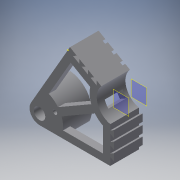
# Autodesk Inventor part: Base_Alpha_V1.1_6mm_
Saved by Autodesk Inventor 2016 (Build 200138000, 138)
## iProperties
Created: 2015-12-07
Part Number: Base_Alpha_V1.1_6mm_
Material: Generic
Document SubType Name: Modeling
Designer: Daniel
Density: 1 g/cm^3
Appearance: Default
Author: Daniel
Autodesk Inventor part; units mm, degrees
ref_plane "YZ Plane" through (0, 0, 0) normal (1, 0, 0) x (0, 1, 0)
ref_plane "XZ Plane" through (0, 0, 0) normal (0, 1, 0) x (-1, 0, 0)
ref_plane "XY Plane" through (0, 0, 0) normal (0, 0, 1) x (1, 0, 0)
sketch "Sketch1" plane through (0, 0, 0) normal (0, 1, 0) x (-1, 0, 0)
  circle A0 centre (103.923, -60) radius 8
  line L0 (24.2487, 14) -> (32.909, 19)
  line L1 (36.3731, 21) -> (45.0333, 26)
  line L2 (48.4974, 28) -> (57.1577, 33)
  line L3 (0, -28) -> (0, -38)
  line L4 (0, -42) -> (0, -52)
  line L5 (0, -56) -> (0, -66)
  line L6 (5.1962, -74) -> (103.923, -74)
  arc A1 (103.923, -74) -> (116.0474, -53) centre (103.923, -60) ccw
  line L7 (116.0474, -53) -> (61.4878, 41.5)
  arc A2 (5.1962, -23.4307) -> (17.6935, 16.2154) centre (0, 0) ccw
  line L8 (5.1962, -23.4307) -> (5.1962, -31)
  line L9 (5.1962, -31) -> (0, -28)
  line L10 (0, -28) -> (0, -38)
  line L11 (0, -38) -> (5.1962, -35)
  line L12 (5.1962, -35) -> (5.1962, -45)
  line L13 (5.1962, -45) -> (0, -42)
  line L14 (0, -42) -> (0, -52)
  line L15 (0, -52) -> (5.1962, -49)
  line L16 (5.1962, -49) -> (5.1962, -59)
  line L17 (5.1962, -59) -> (0, -56)
  line L18 (0, -56) -> (0, -66)
  line L19 (0, -66) -> (5.1962, -63)
  line L20 (5.1962, -63) -> (5.1962, -74)
  line L21 (17.6935, 16.2154) -> (24.2487, 20)
  line L22 (24.2487, 20) -> (24.2487, 14)
  line L23 (24.2487, 14) -> (32.909, 19)
  line L24 (32.909, 19) -> (27.7128, 22)
  line L25 (27.7128, 22) -> (36.3731, 27)
  line L26 (36.3731, 27) -> (36.3731, 21)
  line L27 (36.3731, 21) -> (45.0333, 26)
  line L28 (45.0333, 26) -> (39.8372, 29)
  line L29 (39.8372, 29) -> (48.4974, 34)
  line L30 (48.4974, 34) -> (48.4974, 28)
  line L31 (48.4974, 28) -> (57.1577, 33)
  line L32 (57.1577, 33) -> (51.9615, 36)
  line L33 (51.9615, 36) -> (61.4878, 41.5)
  line L34 (91.0088, -29.6319) -> (60.4256, 23.3397)
  line L35 (60.4256, 23.3397) -> (33.1425, 7.5878)
  arc A3 (31.6247, -12.485) -> (33.1425, 7.5878) centre (0, 0) ccw
  line L36 (31.6247, -12.485) -> (78.1742, -39.3604)
  arc A4 (91.0088, -29.6319) -> (78.1742, -39.3604) centre (103.923, -60) ccw
  line L37 (71.1664, -64) -> (15.1962, -64)
  line L38 (15.1962, -64) -> (15.1962, -30.4151)
  arc A5 (15.1962, -30.4151) -> (26.6247, -21.1453) centre (0, 0) ccw
  line L39 (26.6247, -21.1453) -> (73.1742, -48.0206)
  arc A6 (73.1742, -48.0206) -> (71.1664, -64) centre (103.923, -60) ccw
  line L40 (61.4878, 41.5) -> (116.0474, -53)
  line L41 (61.4878, 41.5) -> (51.9615, 36)
  line L42 (57.1577, 33) -> (51.9615, 36)
  line L43 (57.1577, 33) -> (48.4974, 28)
  line L44 (48.4974, 34) -> (48.4974, 28)
  line L45 (48.4974, 34) -> (39.8372, 29)
  line L46 (45.0333, 26) -> (39.8372, 29)
  line L47 (45.0333, 26) -> (36.3731, 21)
  line L48 (36.3731, 21) -> (36.3731, 27)
  line L49 (36.3731, 27) -> (27.7128, 22)
  line L50 (32.909, 19) -> (27.7128, 22)
  line L51 (32.909, 19) -> (24.2487, 14)
  line L52 (24.2487, 14) -> (24.2487, 20)
  line L53 (24.2487, 20) -> (17.6935, 16.2154)
  line L54 (5.1962, -23.4307) -> (5.1962, -31)
  line L55 (0, -28) -> (5.1962, -31)
  line L56 (0, -28) -> (0, -38)
  line L57 (5.1962, -35) -> (0, -38)
  line L58 (5.1962, -35) -> (5.1962, -45)
  line L59 (0, -42) -> (5.1962, -45)
  line L60 (0, -42) -> (0, -52)
  line L61 (0, -52) -> (5.1962, -49)
  line L62 (5.1962, -49) -> (5.1962, -59)
  line L63 (0, -56) -> (5.1962, -59)
  line L64 (0, -56) -> (0, -66)
  line L65 (5.1962, -63) -> (0, -66)
  line L66 (5.1962, -63) -> (5.1962, -74)
  line L67 (5.1962, -74) -> (103.923, -74)
  line L68 (71.1664, -64) -> (15.1962, -64)
  line L69 (15.1962, -64) -> (15.1962, -30.4151)
  line L70 (26.6247, -21.1453) -> (73.1742, -48.0206)
  line L71 (31.6247, -12.485) -> (78.1742, -39.3604)
  line L72 (33.1425, 7.5878) -> (60.4256, 23.3397)
  line L73 (60.4256, 23.3397) -> (91.0088, -29.6319)
  arc A7 (31.6247, -12.485) -> (33.1425, 7.5878) centre (0, 0) ccw
  arc A8 (15.1962, -30.4151) -> (26.6247, -21.1453) centre (0, 0) ccw
  arc A9 (73.1742, -48.0206) -> (71.1664, -64) centre (103.923, -60) ccw
  arc A10 (91.0088, -29.6319) -> (78.1742, -39.3604) centre (103.923, -60) ccw
  arc A11 (5.1962, -23.4307) -> (17.6935, 16.2154) centre (0, 0) ccw
  arc A12 (103.923, -74) -> (116.0474, -53) centre (103.923, -60) ccw
  circle A13 centre (103.923, -60) radius 8
  circle A14 centre (82.2724, -47.5) radius 3
  point P0 (0, 0)
  dimension "d38" = 6
  dimension "d39" = 25
  constraints: 148 end point, 24 point on circle, 22 collinear, 15 centre point, 9 parallel, 6 point on line, 4 concentric, 2 perpendicular, 2 tangent, 1 coincident
  measures "d38" diameter of A14
  measures "d39" distance of A0.centre A14.centre
ref_plane "Plano de trabajo1" through (0, 10, 0) normal (0, 1, 0) x (1, 0, 0)
sketch "Boceto2" plane through (0, 10, 0) normal (0, 1, 0) x (1, 0, 0)
  arc A0 (-103.923, 74) -> (-116.0474, 53) centre (-103.923, 60) ccw
  circle A1 centre (-103.923, 60) radius 8 projected
  arc A2 (-101.1059, 27.1205) -> (-74.0399, 74) centre (-103.923, 60) ccw
  line L0 (-103.923, 74) -> (-74.0399, 74)
  arc A3 (-73.1742, 48.0206) -> (-71.1664, 64) centre (-103.923, 60) ccw projected
  arc A4 (-103.923, 74) -> (-116.0474, 53) centre (-103.923, 60) ccw projected
  line L1 (-116.0474, 53) -> (-101.1059, 27.1205)
  circle A5 centre (-103.923, 60) radius 8
  circle A6 centre (-82.2724, 47.5) radius 3
  line L2 (-31.6247, 12.485) -> (-22.8286, 7.4066)
  arc A7 (-31.6247, 12.485) -> (-31.5514, -12.6692) centre (0, 0) ccw
  line L3 (-27.7128, -22) -> (-32.909, -19) projected
  line L4 (-32.909, -19) -> (-27.7128, -22)
  line L5 (-36.3731, -21) -> (-36.3731, -27) projected
  line L6 (-27.7128, -22) -> (-36.3731, -27)
  line L7 (-36.3731, -27) -> (-36.3731, -21)
  line L8 (-45.0333, -26) -> (-39.8372, -29)
  line L9 (-48.4974, -34) -> (-39.8372, -29) projected
  line L10 (-39.8372, -29) -> (-48.4974, -34)
  line L11 (-48.4974, -34) -> (-48.4974, -28)
  line L12 (-51.9615, -36) -> (-57.1577, -33) projected
  line L13 (-57.1577, -33) -> (-51.9615, -36)
  line L14 (-51.9615, -36) -> (-61.4878, -41.5)
  line L15 (-24.2487, -14) -> (-24.2487, -20) projected
  line L16 (-24.2487, -20) -> (-17.6935, -16.2154)
  line L17 (-24.2487, -14) -> (-24.2487, -20) projected
  line L18 (-24.2487, -14) -> (-24.2487, -20)
  line L19 (-24.2487, -14) -> (-29.4449, -17)
  line L20 (-78.1742, 39.3604) -> (-31.6247, 12.485) projected
  arc A8 (-5.1962, 23.4307) -> (-17.6935, -16.2154) centre (0, 0) ccw projected
  arc A9 (-22.8286, 7.4066) -> (-17.6935, -16.2154) centre (0, 0) ccw
  line L21 (0, 28) -> (0, 38) projected
  line L22 (0, 28) -> (0, 38)
  line L23 (-5.1962, 35) -> (-5.1962, 45) projected
  line L24 (0, 38) -> (-5.1962, 35)
  line L25 (0, 38) -> (-5.1962, 35) projected
  line L26 (-5.1962, 31) -> (0, 28) projected
  line L27 (-5.1962, 31) -> (0, 28)
  line L28 (-5.1962, 45) -> (0, 42) projected
  line L29 (0, 42) -> (-5.1962, 45)
  line L30 (0, 52) -> (-5.1962, 49) projected
  line L31 (-5.1962, 49) -> (0, 52)
  line L32 (0, 52) -> (0, 42)
  line L33 (0, 42) -> (0, 52) projected
  line L34 (0, 56) -> (0, 66) projected
  line L35 (0, 56) -> (0, 66)
  line L36 (0, 66) -> (-5.1962, 63) projected
  line L37 (0, 66) -> (-5.1962, 63)
  line L38 (-5.1962, 49) -> (-5.1962, 59) projected
  line L39 (-5.1962, 59) -> (0, 56)
  arc A10 (-5.1962, 23.4307) -> (-17.6935, -16.2154) centre (0, 0) ccw projected
  line L40 (-26.6247, 21.1453) -> (-17.8286, 16.0668)
  arc A11 (-5.1962, 23.4307) -> (-17.8286, 16.0668) centre (0, 0) ccw
  line L41 (-5.1962, 23.4307) -> (-5.1962, 31)
  line L42 (-61.4878, -41.5) -> (-66.4878, -32.8397)
  line L43 (-116.0474, 53) -> (-61.4878, -41.5) projected
  line L44 (-66.4878, -32.8397) -> (-31.5514, -12.6692)
  line L45 (-27.7128, -22) -> (-32.909, -19) projected
  line L46 (-32.909, -19) -> (-29.4449, -17)
  line L47 (-32.909, -19) -> (-24.2487, -14) projected
  line L48 (-57.1577, -33) -> (-48.4974, -28) projected
  line L49 (-57.1577, -33) -> (-48.4974, -28)
  line L50 (-45.0333, -26) -> (-36.3731, -21)
  line L51 (-5.1962, 74) -> (-103.923, 74) projected
  line L52 (-5.1962, 74) -> (-10.1962, 74)
  line L53 (-15.1962, 64) -> (-15.1962, 30.4151) projected
  line L54 (-10.1962, 74) -> (-10.1962, 32.4351)
  line L55 (0, 38) -> (-5.1962, 35) projected
  line L56 (-5.1962, 35) -> (-5.1962, 45)
  line L57 (-5.1962, 49) -> (-5.1962, 59) projected
  line L58 (-5.1962, 59) -> (0, 56) projected
  line L59 (-5.1962, 49) -> (-5.1962, 59)
  line L60 (0, 66) -> (-5.1962, 63) projected
  line L61 (-5.1962, 63) -> (-5.1962, 74) projected
  line L62 (-5.1962, 63) -> (-5.1962, 74)
  arc A12 (-15.1962, 30.4151) -> (-26.6247, 21.1453) centre (0, 0) ccw projected
  arc A13 (-10.1962, 32.4351) -> (-26.6247, 21.1453) centre (0, 0) ccw
  line L63 (-103.923, 60) -> (0, 0) construction
  point P0 (0, 0)
  dimension "d33" = 10
  dimension "d34" = 5
  dimension "d42" = 6
  dimension "d43" = 30
  dimension "d44" = 29.4449
  constraints: 72 end point, 16 collinear, 15 point on circle, 8 centre point, 8 coincident, 5 parallel, 3 point on line, 2 vertical, 1 concentric, 1 tangent
  measures "d33" distance of L14.end L42.end
  measures "d34" distance of L51.start L52.end
  measures "d42" diameter of A6
  measures "d43" angle of L36 L0
  measures "d44" distance from line of L19.end L21
ref_plane "Plano de trabajo2" through (0, 35, 0) normal (0, 1, 0) x (1, 0, 0)
sketch "Boceto4" plane through (0, 35, 0) normal (0, 1, 0) x (1, 0, 0)
  arc A0 (-101.1059, 27.1205) -> (-74.0399, 74) centre (-103.923, 60) ccw
  arc A1 (-103.923, 74) -> (-116.0474, 53) centre (-103.923, 60) ccw
  line L0 (-116.0474, 53) -> (-101.1059, 27.1205)
  line L1 (-116.0474, 53) -> (-101.1059, 27.1205) projected
  line L2 (-74.0399, 74) -> (-103.923, 74) projected
  arc A2 (-103.923, 74) -> (-116.0474, 53) centre (-103.923, 60) ccw projected
  line L3 (-74.0399, 74) -> (-103.923, 74)
  line L4 (-5.1962, 35) -> (0, 38)
  line L5 (-5.1962, 31) -> (0, 28) projected
  line L6 (0, 38) -> (0, 28)
  line L7 (0, 28) -> (-5.1962, 31)
  line L8 (-5.1962, 23.4307) -> (-5.1962, 31) projected
  line L9 (-5.1962, 31) -> (-5.1962, 23.4307)
  line L10 (-29.4449, -17) -> (-24.2487, -14)
  line L11 (-24.2487, -14) -> (-24.2487, -20) projected
  line L12 (-24.2487, -14) -> (-24.2487, -20)
  line L13 (-24.2487, -20) -> (-17.6935, -16.2154) projected
  line L14 (-24.2487, -20) -> (-17.6935, -16.2154)
  arc A3 (-5.1962, 23.4307) -> (-5.1962, 23.4307) centre (0, 0) ccw
  line L15 (-61.4878, -41.5) -> (-51.9615, -36) projected
  line L16 (-48.4974, -28) -> (-48.4974, -34) projected
  line L17 (-39.8372, -29) -> (-45.0333, -26) projected
  line L18 (-36.3731, -21) -> (-36.3731, -27) projected
  line L19 (-36.3731, -27) -> (-27.7128, -22) projected
  line L20 (-27.7128, -22) -> (-32.909, -19) projected
  line L21 (-5.1962, 45) -> (0, 42) projected
  line L22 (0, 42) -> (0, 52) projected
  line L23 (0, 52) -> (-5.1962, 49) projected
  line L24 (-10.1962, 74) -> (-10.1962, 32.4351) projected
  arc A4 (-5.1962, 23.4307) -> (-17.8286, 16.0668) centre (0, 0) ccw projected
  line L25 (-5.1962, 23.4307) -> (-5.1962, 31) projected
  line L26 (-5.1962, 31) -> (0, 28) projected
  line L27 (0, 28) -> (0, 38) projected
  line L28 (-5.1962, 63) -> (-5.1962, 74) projected
  line L29 (-5.1962, 74) -> (-10.1962, 74) projected
  line L30 (0, 38) -> (-5.1962, 35) projected
  line L31 (-5.1962, 35) -> (-5.1962, 45) projected
  line L32 (-5.1962, 45) -> (0, 42) projected
  line L33 (0, 42) -> (0, 52) projected
  line L34 (0, 52) -> (-5.1962, 49) projected
  line L35 (-5.1962, 49) -> (-5.1962, 59) projected
  line L36 (-5.1962, 59) -> (0, 56) projected
  line L37 (0, 56) -> (0, 66) projected
  line L38 (0, 66) -> (-5.1962, 63) projected
  line L39 (-10.1962, 74) -> (-10.1962, 32.4351) projected
  line L40 (-26.6247, 21.1453) -> (-17.8286, 16.0668)
  arc A5 (-5.1962, 23.4307) -> (-17.8286, 16.0668) centre (0, 0) ccw projected
  line L41 (-5.1962, 23.4307) -> (-5.1962, 31) projected
  line L42 (-5.1962, 31) -> (0, 28) projected
  line L43 (0, 28) -> (0, 38) projected
  line L44 (0, 38) -> (-5.1962, 35) projected
  line L45 (-5.1962, 35) -> (-5.1962, 45) projected
  line L46 (-5.1962, 49) -> (-5.1962, 59) projected
  line L47 (-5.1962, 59) -> (0, 56) projected
  line L48 (0, 56) -> (0, 66) projected
  line L49 (0, 66) -> (-5.1962, 63) projected
  line L50 (-5.1962, 63) -> (-5.1962, 74) projected
  line L51 (-5.1962, 74) -> (-10.1962, 74) projected
  line L52 (-31.5514, -12.6692) -> (-66.4878, -32.8397) projected
  line L53 (-66.4878, -32.8397) -> (-61.4878, -41.5) projected
  line L54 (-61.4878, -41.5) -> (-51.9615, -36) projected
  line L55 (-51.9615, -36) -> (-57.1577, -33) projected
  line L56 (-57.1577, -33) -> (-48.4974, -28) projected
  line L57 (-48.4974, -28) -> (-48.4974, -34) projected
  line L58 (-48.4974, -34) -> (-39.8372, -29) projected
  line L59 (-39.8372, -29) -> (-45.0333, -26) projected
  line L60 (-45.0333, -26) -> (-36.3731, -21) projected
  line L61 (-36.3731, -21) -> (-36.3731, -27) projected
  line L62 (-32.909, -19) -> (-24.2487, -14) projected
  line L63 (-24.2487, -14) -> (-24.2487, -20) projected
  line L64 (-24.2487, -20) -> (-17.6935, -16.2154) projected
  line L65 (-31.5514, -12.6692) -> (-66.4878, -32.8397) projected
  line L66 (-66.4878, -32.8397) -> (-61.4878, -41.5) projected
  line L67 (-61.4878, -41.5) -> (-51.9615, -36) projected
  line L68 (-51.9615, -36) -> (-57.1577, -33) projected
  line L69 (-57.1577, -33) -> (-48.4974, -28) projected
  line L70 (-48.4974, -34) -> (-39.8372, -29) projected
  line L71 (-45.0333, -26) -> (-36.3731, -21) projected
  line L72 (-36.3731, -21) -> (-36.3731, -27) projected
  line L73 (-36.3731, -27) -> (-27.7128, -22) projected
  line L74 (-27.7128, -22) -> (-32.909, -19) projected
  line L75 (-32.909, -19) -> (-24.2487, -14) projected
  line L76 (-24.2487, -14) -> (-24.2487, -20) projected
  line L77 (-24.2487, -20) -> (-17.6935, -16.2154) projected
  arc A6 (-31.6247, 12.485) -> (-31.5514, -12.6692) centre (0, 0) ccw projected
  line L78 (-31.5514, -12.6692) -> (-66.4878, -32.8397) projected
  line L79 (-66.4878, -32.8397) -> (-61.4878, -41.5) projected
  line L80 (-51.9615, -36) -> (-57.1577, -33) projected
  line L81 (-57.1577, -33) -> (-48.4974, -28) projected
  line L82 (-48.4974, -28) -> (-48.4974, -34) projected
  line L83 (-48.4974, -34) -> (-39.8372, -29) projected
  line L84 (-39.8372, -29) -> (-45.0333, -26) projected
  line L85 (-45.0333, -26) -> (-36.3731, -21) projected
  line L86 (-36.3731, -21) -> (-36.3731, -27) projected
  line L87 (-36.3731, -27) -> (-27.7128, -22) projected
  line L88 (-27.7128, -22) -> (-32.909, -19) projected
  line L89 (-32.909, -19) -> (-24.2487, -14) projected
  line L90 (-24.2487, -14) -> (-24.2487, -20) projected
  line L91 (-24.2487, -20) -> (-17.6935, -16.2154) projected
  arc A7 (-22.8286, 7.4066) -> (-17.6935, -16.2154) centre (0, 0) ccw projected
  arc A8 (-10.1962, 32.4351) -> (-26.6247, 21.1453) centre (0, 0) ccw projected
  arc A9 (-10.1962, 32.4351) -> (-26.6247, 21.1453) centre (0, 0) ccw projected
  arc A10 (-31.6247, 12.485) -> (-31.5514, -12.6692) centre (0, 0) ccw
  arc A11 (-22.8286, 7.4066) -> (-17.6935, -16.2154) centre (0, 0) ccw
  line L92 (-26.6247, 21.1453) -> (-17.8286, 16.0668)
  arc A12 (-10.1962, 32.4351) -> (-26.6247, 21.1453) centre (0, 0) ccw projected
  line L93 (-17.8286, 16.0668) -> (-26.6247, 21.1453)
  arc A13 (-10.1962, 32.4351) -> (-31.5514, -12.6692) centre (0, 0) ccw
  arc A14 (-5.1962, 23.4307) -> (-17.6935, -16.2154) centre (0, 0) ccw
  point P0 (0, 0)
  point P1 (-20.7846, -12)
  point P2 (-61.4878, -41.5)
  point P3 (-52.8275, -36.5)
  point P4 (-39.3157, 16.9254)
  constraints: 25 end point, 14 point on circle, 13 centre point, 7 coincident, 5 collinear, 1 horizontal, 1 tangent, 2 other
extrude "Extrusión6" add sketch "Sketch1" along normal blind 10
extrude "Extrusión7" add sketch "Boceto2" along normal blind 25 contours L0 A2 L1 A0 | L51 L61 L36 L34 L39 L38 L30 L32 L28 L23 L24 L21 L26 L41 A8 L40 A12 A13 L54 | L44 A7 L2 A8 L16 L15 L19 L46 L3 L6 L5 L50 L8 L9 L11 L48 L12 L14 L42
extrude "Extrusión8" add sketch "Boceto4" along normal blind 5 contours L0 A1 L2 A0 | L4 L6 L5 L8 A3 L40 A8 L24 L29 L28 L38 L37 L36 L35 L23 L22 L21 L31 | A3 L13 L11 L10 L62 L20 L19 L18 L60 L17 L58 L16 L56 L55 L15 L53 L52 A6 A13 L40
sketch "Boceto7" plane through (-61.4878, 0, 41.5) normal (-0.8660254, 0, 0.5) x (0.5, 0, 0.8660254)
  point P0 (-5.1962, 0)
